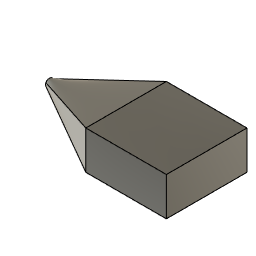
CFD mesh v1 (Autodesk Fusion 360 design; units mm, degrees)
Autodesk Fusion 360 part; units mm, degrees
sketch "Sketch1" plane through (0, 0, 0) normal (0, 0, 1) x (1, 0, 0)
  line L0 (0, 0) -> (210, 0)
  line L1 (210, 0) -> (210, 210)
  line L2 (210, 210) -> (0, 210)
  line L3 (0, 210) -> (0, 0)
  dimension "d1" = 210
  dimension "d2" = 210
  constraint horizontal L0
  constraint vertical L1
  constraint horizontal L2
  constraint vertical L3
  constraint coincident L0.start L3.end
  measures "d1" distance of L0.start L0.end
  measures "d2" distance of L0.start L2.end
extrude "Extrude1" add sketch "Sketch1" along normal blind 100
ref_plane "WorkPlane1" through (-200, 105, 50) normal (-1, 0, 0) x (0, -1, 0)
sketch "Sketch2" plane through (-200, 105, 50) normal (-1, 0, 0) x (0, 1, 0)
  circle A0 centre (0, 0) radius 10
  dimension "d6" = 20
  constraint coincident A0.centre origin
  measures "d6" diameter of A0
loft "Loft1" add profiles "Sketch2" section 1 face at (0, 140, 33.3333) section 2
